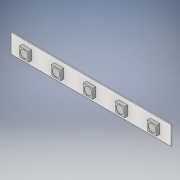
# Autodesk Inventor part: LED Strip 5050 x 5
Saved by Autodesk Inventor 2019 (Build 230136000, 136)
## iProperties
Created: 2021-08-04
Part Number: LED Strip 5050 x 5
Material: Generic
Document SubType Name: Modeling
Designer: Lix
Density: 1 g/cm^3
Appearance: Default
Author: Lix
Autodesk Inventor part; units mm, degrees
ref_plane "YZ Plane" through (0, 0, 0) normal (1, 0, 0) x (0, 1, 0)
ref_plane "XZ Plane" through (0, 0, 0) normal (0, 1, 0) x (-1, 0, 0)
ref_plane "XY Plane" through (0, 0, 0) normal (0, 0, 1) x (1, 0, 0)
sketch "Sketch1" plane through (0, 0, 0) normal (0, 0, 1) x (1, 0, 0)
  line L0 (-42.5, 5) -> (42.5, 5)
  line L1 (42.5, 5) -> (42.5, -5)
  line L2 (42.5, -5) -> (-42.5, -5)
  line L3 (-42.5, -5) -> (-42.5, 5)
  line L4 (-42.5, 5) -> (42.5, -5) construction
  line L5 (42.5, 5) -> (-42.5, -5) construction
  point P0 (0, 0)
  dimension "d0" = 85
  dimension "d1" = 10
  constraints: 12 end point, 2 midpoint, 2 parallel, 1 horizontal, 1 perpendicular
  measures "d0" distance of L1.end L2.end
  measures "d1" distance of L0.end L1.end
extrude "Extrusion1" add sketch "Sketch1" along normal blind 0.5
sketch "Sketch2" plane through (0, 0, 0.5) normal (0, 0, 1) x (1, 0, 0)
  line L0 (-36.5, 2.5) -> (-31.5, 2.5)
  line L1 (-31.5, 2.5) -> (-31.5, -2.5)
  line L2 (-31.5, -2.5) -> (-36.5, -2.5)
  line L3 (-36.5, -2.5) -> (-36.5, 2.5)
  line L4 (-36.5, 2.5) -> (-31.5, -2.5) construction
  line L5 (-31.5, 2.5) -> (-36.5, -2.5) construction
  line L6 (-42.5, 5) -> (-42.5, -5) projected
  point P0 (0, 0)
  point P1 (-34, 0)
  point P2 (-34, 0)
  point P3 (-42.5, 0)
  dimension "d4" = 5
  dimension "d5" = 5
  dimension "d6" = 6
  constraints: 12 end point, 4 midpoint, 2 parallel, 1 horizontal, 1 horizontal alignment, 1 perpendicular
  measures "d4" distance of L1.end L2.end
  measures "d5" distance of L0.end L1.end
  measures "d6" distance between parallel lines of L3 L6
extrude "Extrusion2" add sketch "Sketch2" along normal blind 1.6
sketch "Sketch3" plane through (0, 0, 2.1) normal (0, 0, 1) x (1, 0, 0)
  line L0 (-31.5, 2.5) -> (-36.5, 2.5) projected
  line L1 (-36.5, 2.5) -> (-36.5, -2.5) projected
  line L2 (-36.5, -2.5) -> (-31.5, -2.5) projected
  line L3 (-31.5, -2.5) -> (-31.5, 2.5) projected
  circle A0 centre (-34, 0) radius 2.05
  point P0 (0, 0)
  point P1 (-31.5, 0)
  point P2 (-34, 2.5)
  dimension "d9" = 4.1
  constraints: 2 midpoint, 1 centre point, 1 horizontal alignment, 1 vertical alignment
  measures "d9" diameter of A0
extrude "Extrusion3" cut sketch "Sketch3" against normal blind 0.1 contours A0
pattern_linear "Rectangular Pattern1" count 5 spacing 17 along (1, 0, 0) of "Extrusion3", "Extrusion2"
body "Solid1"
